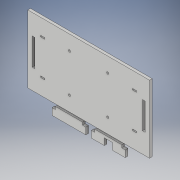
# Autodesk Inventor part: mount - developer
Saved by Autodesk Inventor 2019 (Build 230136000, 136)
## iProperties
Created: 2019-04-11
Part Number: mount - developer
Material: Generic
Document SubType Name: Modeling
Designer: jonas
Density: 1 g/cm^3
Appearance: Default
Author: jonas
Autodesk Inventor part; units mm, degrees
ref_plane "YZ Plane" through (0, 0, 0) normal (1, 0, 0) x (0, 1, 0)
ref_plane "XZ Plane" through (0, 0, 0) normal (0, 1, 0) x (-1, 0, 0)
ref_plane "XY Plane" through (0, 0, 0) normal (0, 0, 1) x (1, 0, 0)
sketch "Sketch1" plane through (0, 0, 0) normal (0, 0, 1) x (1, 0, 0)
  line L0 (-90, -50) -> (90, -50)
  line L1 (90, -50) -> (90, 50)
  line L2 (90, 50) -> (-90, 50)
  line L3 (-90, 50) -> (-90, -50)
  line L4 (0, 1.1499) -> (0, -1.1499)
  line L5 (1.5253, 0) -> (-2.0225, 0)
  line L6 (-83.5, -20) -> (-79.5, -20)
  line L7 (-79.5, -20) -> (-79.5, 20)
  line L8 (-79.5, 20) -> (-83.5, 20)
  line L9 (-83.5, 20) -> (-83.5, -20)
  line L10 (83.5, -20) -> (79.5, -20)
  line L11 (79.5, -20) -> (79.5, 20)
  line L12 (79.5, 20) -> (83.5, 20)
  line L13 (83.5, 20) -> (83.5, -20)
  line L14 (-4.1143, -67.1712) -> (-4.1143, -57.1712)
  line L15 (-4.1143, -57.1712) -> (-9.1143, -57.1712)
  line L16 (-54.1143, -57.1712) -> (-54.1143, -67.1712)
  line L17 (-54.1143, -67.1712) -> (-4.1143, -67.1712)
  line L18 (-49.1143, -53.1712) -> (-9.1143, -53.1712)
  line L19 (-9.1143, -53.1712) -> (-9.1143, -57.1712)
  line L20 (-49.1143, -57.1712) -> (-54.1143, -57.1712)
  line L21 (-49.1143, -57.1712) -> (-49.1143, -53.1712)
  circle A0 centre (-28.2843, -28.2843) radius 1.6
  circle A1 centre (28.2843, -28.2843) radius 1.6
  circle A2 centre (28.2843, 28.2843) radius 1.6
  circle A3 centre (-28.2843, 28.2843) radius 1.6
  line L22 (0, 0) -> (3.5355, -3.5355)
  line L23 (0, 0) -> (5, 0) construction
  line L24 (4.1143, -67.1712) -> (4.1143, -57.1712)
  line L25 (4.1143, -57.1712) -> (9.1143, -57.1712)
  line L26 (54.1143, -57.1712) -> (54.1143, -67.1712)
  line L27 (54.1143, -67.1712) -> (35.1143, -67.1712)
  line L28 (49.1143, -53.1712) -> (9.1143, -53.1712)
  line L29 (9.1143, -53.1712) -> (9.1143, -57.1712)
  line L30 (49.1143, -57.1712) -> (54.1143, -57.1712)
  line L31 (49.1143, -57.1712) -> (49.1143, -53.1712)
  line L32 (35.1143, -57.1712) -> (23.1143, -57.1712)
  line L33 (23.1143, -57.1712) -> (23.1143, -67.1712)
  line L34 (23.1143, -67.1712) -> (4.1143, -67.1712)
  line L35 (35.1143, -67.1712) -> (35.1143, -57.1712)
  line L36 (-71, 27) -> (-65, 27)
  line L37 (-65, 27) -> (-65, 25)
  line L38 (-65, 25) -> (-71, 25)
  line L39 (-71, 25) -> (-71, 27)
  line L40 (71, 27) -> (65, 27)
  line L41 (65, 27) -> (65, 25)
  line L42 (65, 25) -> (71, 25)
  line L43 (71, 25) -> (71, 27)
  line L44 (-71, -27) -> (-65, -27)
  line L45 (-65, -27) -> (-65, -25)
  line L46 (-65, -25) -> (-71, -25)
  line L47 (-71, -25) -> (-71, -27)
  line L48 (65, -27) -> (65, -25)
  line L49 (71, -27) -> (65, -27)
  line L50 (71, -25) -> (71, -27)
  line L51 (65, -25) -> (71, -25)
  dimension "d0" = 100
  dimension "d1" = 180
  dimension "d2" = 159
  dimension "d3" = 40
  dimension "d4" = 4
  dimension "d6" = 5
  dimension "d7" = 10
  dimension "d8" = 3.2
  dimension "d11" = 360
  dimension "d14" = 4
  dimension "d16" = 45
  dimension "d17" = 40
  dimension "d18" = 50
  dimension "d19" = 5
  dimension "d20" = 4
  dimension "d24" = 6
  dimension "d25" = 2
  dimension "d26" = 25
  dimension "d27" = 65
  constraints: 104 end point, 24 symmetric about line, 11 parallel, 6 perpendicular, 5 horizontal, 4 centre point, 2 midpoint, 2 point on line, 1 collinear, 1 equal length, 1 vertical, 13 other
  measures "d0" distance of L0.end L1.end
  measures "d1" distance of L0.start L0.end
  measures "d2" distance between parallel lines of L11 L7
  measures "d3" distance of L8.end L6.start
  measures "d4" distance of L6.start L6.end
  measures "d6" distance of L14.end L15.end
  measures "d7" distance of L16.start L16.end
  measures "d8" diameter of A0
  measures "d14" distance of L20.start L18.start
  measures "d16" angle of L22 L23
  measures "d17" distance from line of A0.centre L22
  measures "d18" distance between parallel lines of L14 L16
  measures "d19" distance of L20.start L16.start
  measures "d20" distance of L18.end L15.end
  measures "d24" distance of L36.start L36.end
  measures "d25" distance of L38.end L36.start
  measures "d26" distance between parallel lines of L5 L38
  measures "d27" distance between parallel lines of L4 L37
extrude "Extrusion1" add sketch "Sketch1" along normal blind 4
equation "\"d14\" = d4"
equation "\"d18\" = d3 + 2 * d6"
body "Solid1"
